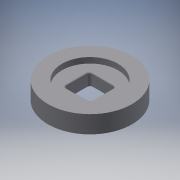
# Autodesk Inventor part: gear_collar_small
Saved by Autodesk Inventor 2019 (Build 230136000, 136)
## iProperties
Created: 2019-01-25
Part Number: gear_collar_small
Material: Generic
Document SubType Name: Modeling
Designer: Varga Daniel
Density: 1 g/cm^3
Appearance: Default
Author: Varga Daniel
Autodesk Inventor part; units mm, degrees
ref_plane "YZ Plane" through (0, 0, 0) normal (1, 0, 0) x (0, 1, 0)
ref_plane "XZ Plane" through (0, 0, 0) normal (0, 1, 0) x (-1, 0, 0)
ref_plane "XY Plane" through (0, 0, 0) normal (0, 0, 1) x (1, 0, 0)
sketch "Sketch1" plane through (0, 0, 0) normal (0, 1, 0) x (-1, 0, 0)
  circle A0 centre (0, 0) radius 6
  dimension "d2" = 12
  constraints: 1 centre point, 1 coincident
  measures "d2" diameter of A0
extrude "Extrusion1" add sketch "Sketch1" along normal blind 2.5
sketch "Sketch2" plane through (0, 2.5, 0) normal (0, 1, 0) x (1, 0, 0)
  line L0 (-1.45, -1.85) -> (1.45, -1.85)
  line L1 (1.85, -1.45) -> (1.85, 1.45)
  line L2 (1.45, 1.85) -> (-1.45, 1.85)
  line L3 (-1.85, 1.45) -> (-1.85, -1.45)
  line L4 (-1.85, -1.85) -> (1.85, 1.85) construction
  line L5 (1.85, -1.85) -> (-1.85, 1.85) construction
  arc A0 (-1.45, 1.85) -> (-1.85, 1.45) centre (-1.45, 1.45) ccw
  arc A1 (-1.85, -1.45) -> (-1.45, -1.85) centre (-1.45, -1.45) ccw
  arc A2 (1.45, -1.85) -> (1.85, -1.45) centre (1.45, -1.45) ccw
  arc A3 (1.85, 1.45) -> (1.45, 1.85) centre (1.45, 1.45) ccw
  point P0 (0, 0)
  dimension "d5" = 3.7
  dimension "d6" = 3.7
  dimension "d7" = 0.4
  constraints: 12 end point, 8 point on circle, 8 point on line, 8 tangent, 4 centre point, 3 equal radius, 2 midpoint, 2 parallel, 1 horizontal, 1 perpendicular
  measures "d5" distance of L5.end L4.end
  measures "d6" distance between parallel lines of L0 L2
  measures "d7" radius of A0
extrude "Extrusion2" cut sketch "Sketch2" against normal through all
sketch "Sketch3" plane through (0, 2.5, 0) normal (0, 1, 0) x (1, 0, 0)
  circle A0 centre (0, 0) radius 4
  dimension "d10" = 8
  constraints: 1 centre point, 1 coincident
  measures "d10" diameter of A0
extrude "Extrusion3" cut sketch "Sketch3" against normal blind 0.8
fillet "Fillet1" radius 0.2 8 edges at (-1.7328, 1.7, 1.7328) (0, 1.7, 1.85) (1.7328, 1.7, 1.7328) (1.85, 1.7, 0) (1.7328, 1.7, -1.7328) (0, 1.7, -1.85) (-1.7328, 1.7, -1.7328) (-1.85, 1.7, 0)
equation "\"d6\" = d5"
body "Solid1"
